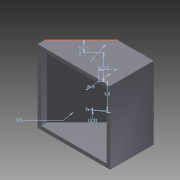
# Autodesk Inventor part: 3039pc4
Saved by Autodesk Inventor 2011 SP1 (Build 150282100, 282)
## iProperties
Company: Allseas Engineering BV
Created: 2011-09-27
Part Number: 3039pc4
Cost Center: 0 kg
Material: Steel
Document SubType Name: Modeling
Designer: BvH
Authority: 0 mm^3
Stock Number: =<Filenr>_<Document number>
Density: 7.85 g/cm^3
Act. Code: DW000
SaveDate: 2011-07-28
SaveTime: 18:32
FileName: Standard
TotalMass: 0 kg
TotalVolume: 0 mm^3
Subject: =<Title><TITLE 1_2> <TITLE 2_2>
Author: BvH
Autodesk Inventor part; units mm, degrees
ref_plane "YZ Plane" through (0, 0, 0) normal (1, 0, 0) x (0, 1, 0)
ref_plane "XZ Plane" through (0, 0, 0) normal (0, 1, 0) x (-1, 0, 0)
ref_plane "XY Plane" through (0, 0, 0) normal (0, 0, 1) x (1, 0, 0)
sketch "Sketch1" plane through (0, 0, 0) normal (0, 0, 1) x (1, 0, 0)
  line L0 (8, 0) -> (-8, 0)
  line L1 (-8, 0) -> (-8, 1.6)
  line L2 (-8, 1.6) -> (0, 9.6)
  line L3 (0, 9.6) -> (8, 9.6)
  line L4 (8, 9.6) -> (8, 0)
  point P0 (0, 0)
  point P1 (0, 0)
  dimension "d0" = 9.6
  dimension "d1" = 16
  dimension "d2" = 8
  dimension "d3" = 1.6
  constraints: 10 end point, 2 horizontal, 2 vertical, 1 coincident, 1 midpoint
  measures "d0" distance between parallel lines of L0 L3
  measures "d1" distance between parallel lines of L4 L1
  measures "d2" distance from line of L2.end L1
  measures "d3" distance of L0.end L1.end
extrude "Extrusion1" add sketch "Sketch1" along normal mid plane 16
shell "Shell1" thickness 0.8 removed faces 1 at (-2.6667, 0, 2.6667)
sketch "Sketch2" plane through (0, 9.6, 8) normal (0, 1, 0) x (1, 0, 0)
  line L0 (4, 12) -> (4, 4) construction
  line L1 (-11.2, 8) -> (11.2, 8) construction
  line L2 (8, 0) -> (8, 16) construction
  circle A0 centre (4, 12) radius 2.5
  circle A1 centre (4, 4) radius 2.5
  point P0 (4, 8)
  dimension "d6" = 4
  dimension "d7" = 8
  dimension "d8" = 5
  constraints: 2 centre point, 2 coincident, 2 end point, 1 equal radius, 1 midpoint, 1 point on line, 1 vertical
  measures "d6" distance between parallel lines of L2 L0
  measures "d7" distance of L0.start L0.end
  measures "d8" diameter of A0
extrude "Extrusion2" add sketch "Sketch2" along normal blind 1.6
sketch "Sketch3" plane through (0, 9.6, -8) normal (-0.7071, 0.7071, 0) x (-0.7071, -0.7071, 0)
  line L0 (11.3137, 16) -> (0, 16) projected
  line L1 (0, 16) -> (0, 0) projected
  line L2 (0, 0) -> (11.3137, 0) projected
  circle A0 centre (3, 2.5) radius 2
  circle A1 centre (3, 8) radius 2.5
  circle A2 centre (3, 13.5) radius 2
  line L3 (4.9365, 14) -> (6.5, 14)
  line L4 (7, 13.5) -> (7, 13.5)
  line L5 (6.5, 13) -> (4.9365, 13)
  line L6 (4.9365, 13) -> (4.9365, 14)
  line L7 (5.4495, 8.5) -> (7.013, 8.5)
  line L8 (7.513, 8) -> (7.513, 8)
  line L9 (7.013, 7.5) -> (5.4495, 7.5)
  line L10 (5.4495, 7.5) -> (5.4495, 8.5)
  line L11 (4.9365, 3) -> (6.5, 3)
  line L12 (7, 2.5) -> (7, 2.5)
  line L13 (6.5, 2) -> (4.9365, 2)
  line L14 (4.9365, 2) -> (4.9365, 3)
  arc A3 (6.5, 2) -> (7, 2.5) centre (6.5, 2.5) ccw
  arc A4 (7, 2.5) -> (6.5, 3) centre (6.5, 2.5) ccw
  arc A5 (7.013, 7.5) -> (7.513, 8) centre (7.013, 8) ccw
  arc A6 (7.513, 8) -> (7.013, 8.5) centre (7.013, 8) ccw
  arc A7 (6.5, 13) -> (7, 13.5) centre (6.5, 13.5) ccw
  arc A8 (7, 13.5) -> (6.5, 14) centre (6.5, 13.5) ccw
  point P0 (6.7882, 8)
  dimension "d12" = 4
  dimension "d13" = 5
  dimension "d14" = 4
  dimension "d15" = 5.5
  dimension "d16" = 5.5
  dimension "d17" = 2.5
  dimension "d18" = 2.5
  dimension "d19" = 3
  dimension "d20" = 0.5
  dimension "d21" = 1
  dimension "d22" = 3.5
  constraints: 24 end point, 18 point on circle, 12 tangent, 10 parallel, 9 centre point, 5 equal radius, 3 horizontal, 3 perpendicular, 2 vertical alignment
  measures "d12" diameter of A2
  measures "d13" diameter of A1
  measures "d14" diameter of A0
  measures "d15" distance of A1.centre A0.centre
  measures "d16" distance of A1.centre A2.centre
  measures "d17" distance from line of L0 A2.centre
  measures "d18" distance from line of L2 A0.centre
  measures "d19" distance from line of L1 A1.centre
  measures "d20" radius of A3
  measures "d21" distance between parallel lines of L5 L3
  measures "d22" distance of A0.centre A3.centre
extrude "Extrusion3" add sketch "Sketch3" along normal blind 0.01
equation "\"d14\" = d12"
equation "\"d16\" = d15"
equation "\"d17\" = d18"
body "Solid1"
